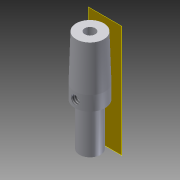
# Autodesk Inventor part: Tool_Mount_Luer_Adapter
Saved by Autodesk Inventor 2011 SP2 (Build 150309200, 309)
## iProperties
Created: 2011-04-26
Part Number: Tool_Mount_Luer_Adapter
Document SubType Name: Modeling
Designer: sungwook
Density: 1.42 g/cm^3
Material: Acetal Resin, White
Mass: 0.375385 g
Surface Area: 4.00827 cm^2
Volume: 0.264355 cm^3
Author: sungwook
Autodesk Inventor part; units mm, degrees
ref_plane "YZ Plane" through (0, 0, 0) normal (1, 0, 0) x (0, 1, 0)
ref_plane "XY Plane" through (0, 0, 0) normal (0, 0, 1) x (1, 0, 0)
sketch "Sketch1" plane through (0, 0, 0) normal (0, 0, 1) x (1, 0, 0)
  circle A0 centre (0, 0) radius 2.159
  dimension "d0" = 4.318
  constraints: 1 centre point, 1 coincident
  measures "d0" diameter of A0
extrude "Extrusion1" add sketch "Sketch1" along normal blind 8.128
sketch "Sketch2" plane through (0, 0, 0) normal (0, 0, -1) x (-1, 0, 0)
  circle A0 centre (0, 0) radius 2.159 projected
  circle A1 centre (0, 0) radius 1.4986
  dimension "d3" = 2.9972
  constraints: 1 centre point, 1 coincident
  measures "d3" diameter of A1
extrude "Extrusion2" cut sketch "Sketch2" against normal blind 6.096
sketch "Sketch3" plane through (0, 0, 0) normal (0, 1, 0) x (-1, 0, 0)
  line L0 (-2.159, 8.128) -> (2.159, 8.128) projected
  line L1 (0, -2.8448) -> (0, 17.0688) projected
  line L2 (2.159, 8.128) -> (0, 8.128)
  line L3 (0, 8.128) -> (0, 14.478)
  line L4 (2.159, 6.096) -> (-2.159, 6.096) projected
  line L5 (-2.159, 8.128) -> (2.159, 8.128) projected
  line L6 (2.159, 6.096) -> (2.159, 8.128) projected
  line L7 (-1.4986, 0) -> (1.4986, 0) projected
  line L8 (0, 14.478) -> (1.9685, 14.478)
  line L9 (1.9685, 14.478) -> (2.159, 8.128)
  point P0 (0, 0)
  dimension "d22" = 8.128
  dimension "d23" = 6.096
  dimension "d24" = 6.35
  dimension "d25" = 1.9685
  constraints: 8 end point, 2 point on line, 1 midpoint, 1 parallel
  measures "d22" distance between parallel lines of L7 L0
  measures "d23" vertical distance of L7.start L4.end
  measures "d24" distance of L2.end L3.end
  measures "d25" distance of L8.end L3.end
revolve "Revolution1" add sketch "Sketch3" angle 360 about axis through (0, 0, -10) along (0, 0, 1) contours L1 L8 L9 L0
hole "Hole1" at (0, 0, 14.478) direction (0, 0, -1) diameter 1.4986 end through all
ref_plane "Work Plane1" through (0, 2.159, 0) normal (0, 1, 0) x (-1, 0, 0)
sketch "Sketch5" plane through (0, 2.159, 0) normal (0, 1, 0) x (-1, 0, 0)
  line L0 (2.159, 6.096) -> (-2.159, 6.096) projected
  line L1 (-2.159, 8.128) -> (2.159, 8.128) projected
  line L2 (0, -2.8956) -> (0, 17.3736) projected
  line L3 (0, 8.128) -> (0, 6.096)
  point P0 (0, 0)
  point P1 (0, 7.112)
  constraints: 3 midpoint, 2 end point, 2 point on line
hole "Hole2" at (0, 2.159, 7.112) direction (0, -1, 0) diameter 1.1938 end through all
equation "\"d25\" = 0.5 * d0 - 0.03 * d6"
equation "\"d6\" = 6.35"
body "Solid1"
